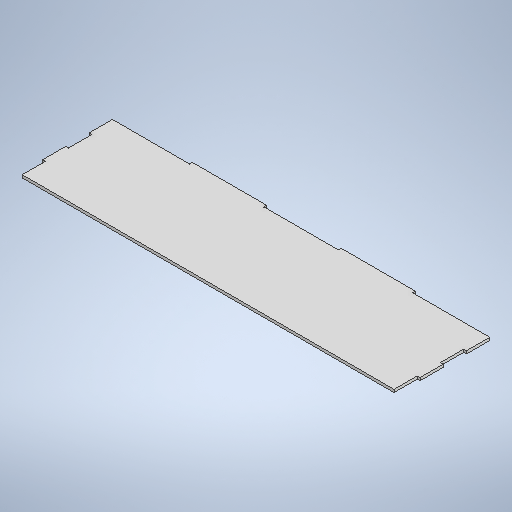
# Autodesk Inventor part: Lateral sup e inf
Saved by Autodesk Inventor 2025.1 (Build 291241020, 241B)
## iProperties
Created: 2024-11-13
Part Number: Lateral sup e inf
Material: Generic
Document SubType Name: Modeling
Designer: marco
Density: 1 g/cm^3
Appearance: Default
Author: marco
Autodesk Inventor part; units mm, degrees
ref_plane "YZ Plane" through (0, 0, 0) normal (1, 0, 0) x (0, 1, 0)
ref_plane "XZ Plane" through (0, 0, 0) normal (0, 1, 0) x (-1, 0, 0)
ref_plane "XY Plane" through (0, 0, 0) normal (0, 0, 1) x (1, 0, 0)
sketch "Sketch1" plane through (0, 0, 0) normal (0, 1, 0) x (-1, 0, 0)
  line L0 (0, 0) -> (400, 0)
  line L1 (400, 0) -> (400, -100)
  line L2 (400, -100) -> (0, -100)
  line L3 (0, -100) -> (0, 0)
  line L4 (320, -103) -> (320, -100)
  line L5 (80, -103) -> (80, -100)
  line L6 (240, -100) -> (240, -103)
  line L7 (160, -103) -> (160, -100)
  line L8 (400, -25) -> (400, -50)
  line L9 (400, -50) -> (403, -50)
  line L10 (200, 0) -> (200, -100) construction
  line L11 (0, 0) -> (0, -100)
  line L12 (-3, -25) -> (0, -25)
  line L13 (0, -25) -> (0, -50)
  line L14 (0, -50) -> (-3, -50)
  line L15 (-3, -75) -> (0, -75)
  line L16 (320, -103) -> (240, -103)
  line L17 (160, -103) -> (80, -103)
  line L18 (0, -100) -> (-3, -100)
  line L19 (-3, -100) -> (-3, -75)
  line L20 (-3, -50) -> (-3, -25)
  line L21 (400, 0) -> (0, 0)
  line L22 (400, -100) -> (400, 0)
  line L23 (403, -75) -> (400, -75)
  line L24 (400, -50) -> (403, -50)
  line L25 (400, -25) -> (400, -50)
  line L26 (403, -25) -> (400, -25)
  line L27 (400, 0) -> (400, -100)
  line L28 (403, -100) -> (403, -75)
  line L29 (403, -50) -> (403, -25)
  line L30 (403, -100) -> (400, -100)
  dimension "d0" = 400
  dimension "d1" = 100
  dimension "d7" = 3
  dimension "d8" = 80
  dimension "d11" = 25
  dimension "d12" = 3
  constraints: 62 end point, 10 point on line, 9 symmetric about line, 5 midpoint, 4 equal length, 4 horizontal, 4 perpendicular
  measures "d0" distance of L1.end L2.end
  measures "d1" distance of L0.end L1.end
  measures "d7" distance of L6.start L6.end
  measures "d8" distance of L6.end L7.start
  measures "d11" distance of L8.start L8.end
  measures "d12" distance of L8.end L9.end
extrude "Extrusion1" add sketch "Sketch1" along normal blind 3
body "Solid1"
